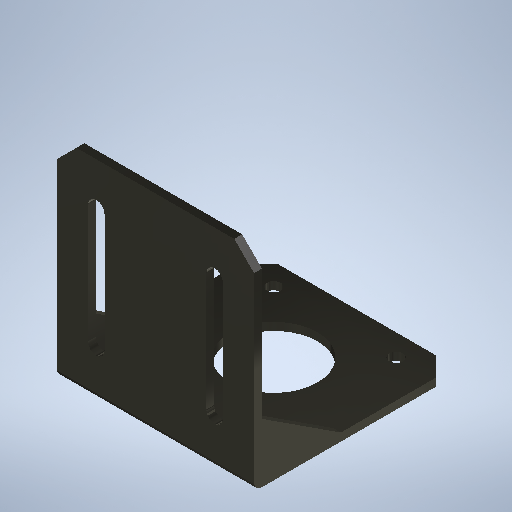
# Autodesk Inventor part: NEMA17Support
Saved by Autodesk Inventor 2026 (Build 300175050, 175E)
## iProperties
Created: 2013-10-13
Part Number: NEMA17Support
Material: Genérico
Document SubType Name: Modeling
Designer: Usuario
Density: 1 g/cm^3
Appearance: Acero - Pulido
Author: Usuario
Autodesk Inventor part; units mm, degrees
ref_plane "YZ Plane" through (0, 0, 0) normal (1, 0, 0) x (0, 1, 0)
ref_plane "XZ Plane" through (0, 0, 0) normal (0, 1, 0) x (-1, 0, 0)
ref_plane "XY Plane" through (0, 0, 0) normal (0, 0, 1) x (1, 0, 0)
sketch "Boceto1" plane through (0, 0, 0) normal (0, 0, 1) x (1, 0, 0)
  line L0 (0, 0) -> (50, 0)
  line L1 (50, 0) -> (50, 46)
  line L2 (45, 51) -> (5, 51)
  line L3 (0, 46) -> (0, 0)
  circle A0 centre (25, 30) radius 11.05
  line L4 (5, 51) -> (0, 46)
  line L5 (50, 46) -> (45, 51)
  point P0 (50, 51)
  point P1 (0, 51)
  point P2 (25, 0)
  point P3 (9.5, 45.5)
  point P4 (40.5, 45.5)
  point P5 (9.5, 14.5)
  point P6 (40.5, 14.5)
  dimension "d0" = 50
  dimension "d1" = 51
  dimension "d2" = 21
  dimension "d3" = 22.1
  dimension "d15" = 5
  dimension "d16" = 5
  dimension "d17" = 5
  dimension "d18" = 5
  dimension "d54" = 31
  dimension "d57" = 31
  dimension "d69" = 21.9203
  constraints: 12 end point, 4 point on line, 2 horizontal, 2 parallel, 1 centre point, 1 midpoint, 1 perpendicular, 1 vertical, 1 vertical alignment, 3 other
  measures "d0" distance of L0.start L0.end
  measures "d1" distance of point (0, 51) L0.start
  measures "d2" distance from line of L2 A0.centre
  measures "d3" diameter of A0
  measures "d15" distance of L2.end point (0, 51)
  measures "d16" distance of L3.start point (0, 51)
  measures "d17" distance of L1.end point (50, 51)
  measures "d18" distance of L2.start point (50, 51)
  measures "d54" distance of point (9.5, 45.5) point (40.5, 45.5)
  measures "d57" distance of point (9.5, 45.5) point (9.5, 14.5)
  measures "d69" distance of A0.centre point (9.5, 45.5)
extrude "Extrusión1" add sketch "Boceto1" along normal blind 2
sketch "Boceto2" plane through (0, 0, 0) normal (0, -1, 0) x (1, 0, 0)
  line L0 (50, 2) -> (0, 2) projected
  line L1 (0, 0) -> (0, 2) projected
  line L2 (0, 0) -> (50, 0) projected
  line L3 (50, 0) -> (50, 2) projected
  line L4 (0, 0) -> (0, 48)
  line L5 (5, 53) -> (45, 53)
  line L6 (50, 48) -> (50, 0)
  line L7 (10, 44.1) -> (10, 44.1)
  line L8 (12.1, 42) -> (12.1, 12)
  line L9 (10, 9.9) -> (10, 9.9)
  line L10 (7.9, 12) -> (7.9, 42)
  arc A0 (10, 44.1) -> (7.9, 42) centre (10, 42) ccw
  arc A1 (12.1, 42) -> (10, 44.1) centre (10, 42) ccw
  arc A2 (7.9, 12) -> (10, 9.9) centre (10, 12) ccw
  arc A3 (10, 9.9) -> (12.1, 12) centre (10, 12) ccw
  line L11 (40, 44.1) -> (40, 44.1)
  line L12 (42.1, 42) -> (42.1, 12)
  line L13 (40, 9.9) -> (40, 9.9)
  line L14 (37.9, 12) -> (37.9, 42)
  arc A4 (40, 44.1) -> (37.9, 42) centre (40, 42) ccw
  arc A5 (42.1, 42) -> (40, 44.1) centre (40, 42) ccw
  arc A6 (37.9, 12) -> (40, 9.9) centre (40, 12) ccw
  arc A7 (40, 9.9) -> (42.1, 12) centre (40, 12) ccw
  line L15 (0, 48) -> (5, 53)
  line L16 (45, 53) -> (50, 48)
  point P0 (0, 53)
  point P1 (50, 53)
  point P2 (7.9, 44.1)
  point P3 (12.1, 44.1)
  point P4 (7.9, 9.9)
  point P5 (37.9, 44.1)
  point P6 (42.1, 44.1)
  point P7 (37.9, 9.9)
  dimension "d21" = 53
  dimension "d24" = 4.2
  dimension "d25" = 7.9
  dimension "d26" = 2.1
  dimension "d27" = 2.1
  dimension "d30" = 30
  dimension "d37" = 5
  dimension "d38" = 5
  dimension "d39" = 5
  dimension "d40" = 5
  dimension "d67" = 30
  dimension "d68" = 11
  constraints: 26 end point, 16 point on circle, 16 point on line, 8 centre point, 8 tangent, 4 parallel, 2 concentric, 2 horizontal, 2 perpendicular, 23 other
  measures "d21" distance of L1.start point (0, 53)
  measures "d24" distance of point (7.9, 44.1) point (12.1, 44.1)
  measures "d25" distance between parallel lines of L4 L10
  measures "d26" radius of A0
  measures "d27" radius of A2
  measures "d30" distance of A0.centre A4.centre
  measures "d37" distance of L4.end point (0, 53)
  measures "d38" distance of L5.start point (0, 53)
  measures "d39" distance of L5.end point (50, 53)
  measures "d40" distance of L6.start point (50, 53)
  measures "d67" distance of A2.centre A0.centre
  measures "d68" vertical distance of A0.centre point (0, 53)
extrude "Extrusión2" add sketch "Boceto2" against normal blind 2 contours L0 L4 L15 L5 L16 L6
sketch "Boceto3" plane through (50, 0, 0) normal (1, 0, 0) x (0, 0, -1)
  line L0 (-2, 46) -> (-2, 2) projected
  line L1 (-2, 2) -> (-48, 2) projected
  line L2 (-2, 2) -> (-2, 22)
  line L3 (-2, 22) -> (-15, 2)
  line L4 (-15, 2) -> (-2, 2)
  dimension "d41" = 20
  dimension "d42" = 13
  constraints: 6 end point, 2 point on line, 1 collinear
  measures "d41" distance of L0.end L2.end
  measures "d42" distance of L0.end L3.end
extrude "Extrusión3" add sketch "Boceto3" against normal blind 2
pattern_linear "Patrón rectangular1" count 2 spacing 48 along (-1, 0, 0) of "Extrusión3"
fillet "Empalme1" radius 2 1 edges at (25, 2, 2)
fillet "Empalme2" radius 2 1 edges at (25, 0, 0)
hole "Hole1" at (9.5, 45.5, 0) at (40.5, 45.5, 0) at (9.5, 14.5, 0) at (40.5, 14.5, 0) direction (0, 0, 1) diameter 3.5 end through all
equation "\"d16\" = d15"
equation "\"d17\" = d15"
equation "\"d18\" = d17"
equation "\"d38\" = d37"
equation "\"d39\" = d37"
equation "\"d40\" = d39"
